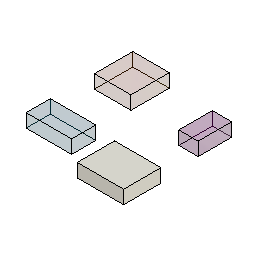
appearance (Autodesk Fusion 360 design; units mm, degrees)
Autodesk Fusion 360 part; units mm, degrees
box "BoxPrimitive1" add length 25.0221 width 14.4211 height 10 placed x (0, 1, 0) y (-1, 0, 0) z (0, 0, 1) at (41.3283, 11.0058, 0) makes body 1
box "BoxPrimitive2" add length 28.6549 width 27.2948 height 10 placed x (0, 1, 0) y (-1, 0, 0) z (0, 0, 1) at (-13.6185, 15.8287, 0) separate body makes body 2
box "BoxPrimitive3" add length 18.0613 width 33.9628 height 10 placed x (0, -1, 0) y (1, 0, 0) z (0, 0, 1) at (-41.2372, -16.6975, 0) separate body makes body 3
box "BoxPrimitive4" add length 27.8473 width 34.617 height 10 placed x (0, -1, 0) y (1, 0, 0) z (0, 0, 1) at (10, -20, 0) separate body makes body 4
named bodies: "MEV", "MF", "Hole", "Key Locator"
